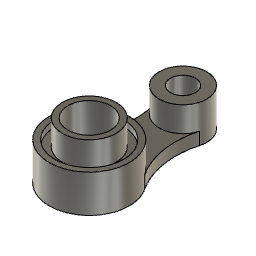
Model 17 (Autodesk Fusion 360 design; units mm, degrees)
Autodesk Fusion 360 part; units mm, degrees
sketch "Sketch1" plane through (0, 0, 0) normal (0, 0, 1) x (1, 0, 0)
  circle A0 centre (0, 0) radius 17
  circle A1 centre (0, 0) radius 21.5
  circle A2 centre (0, 0) radius 27.5
  circle A3 centre (0, 0) radius 32
  line L0 (0, 0) -> (0, 75) construction
  circle A4 centre (0, 75) radius 10
  circle A5 centre (0, 75) radius 19
  arc A6 (-26.678303, 17.671111) -> (-18.321244, 69.966908) centre (-80.034908, 53.013333) ccw
  arc A7 (18.321244, 69.966908) -> (26.678303, 17.671111) centre (80.034908, 53.013333) ccw
  dimension "d1" = 34
  dimension "d2" = 43
  dimension "d3" = 55
  dimension "d4" = 64
  dimension "d5" = 75
  dimension "d6" = 20
  dimension "d7" = 38
  dimension "d8" = 128
  dimension "d9" = 128
  constraint coincident A0.centre A1.centre
  constraint concentric A0 A1
  constraint concentric A1 A3
  constraint vertical L0
  constraint coincident L0.end A4.centre
  constraint concentric A4 A5
  constraint tangent A5 A6
  constraint tangent A3 A6
  constraint tangent A5 A7
  constraint tangent A3 A7
  measures "d1" diameter of A0
  measures "d2" diameter of A1
  measures "d3" diameter of A2
  measures "d4" diameter of A3
  measures "d5" distance of A0.centre L0.end
  measures "d6" diameter of A4
  measures "d7" diameter of A5
  measures "d8" diameter of A7
  measures "d9" diameter of A6
extrude "Extrude1" add sketch "Sketch1" along normal blind 45 contours A1 picked at (19.856662, -1.912709) makes body 1
extrude "Extrude2" add sketch "Sketch1" along normal blind 30 separate body contours A5 picked at (-15.691084, 72.068246) makes body 2
extrude "Extrude3" add sketch "Sketch1" along normal blind 10 contours A3 A5 A6 A7 picked at (8.022936, 43.598649) bodies 2
extrude "Extrude4" add sketch "Sketch1" along normal blind 30 contours A3 picked at (-26.820598, 14.371992) bodies 2
extrude "Extrude5" add sketch "Sketch1" along normal blind 25 contours A2 picked at (25.31757, -2.434357) bodies 1 2
ref_plane "WorkPlane1" through (-16.034908, 53.013333, 5.865013) normal (-1, 0, 0) x (0, 1, 0)
sketch "Sketch2" plane through (-16.034908, 53.013333, 5.865013) normal (-1, 0, 0) x (0, 1, 0)
  line L0 (17.271401, 3.15477) -> (-19.188753, 3.767021) construction
  line L1 (-19.188753, 3.767021) -> (-19.271401, -1.15477) construction
  line L2 (-19.271401, -1.15477) -> (17.188753, -1.767021) construction
  line L3 (17.188753, -1.767021) -> (17.271401, 3.15477) construction
  text T0 "enes şahin" font "Arial" height 5 align left top in box 36.465294 x 4.922485 at (17.271401, 3.15477) x (-0.99985904, 0.01678998) y (-0.01678998, -0.99985904) spacing 1
extrude "Extrude6" add sketch "Sketch2" along normal blind 4 text T0 bodies 1
